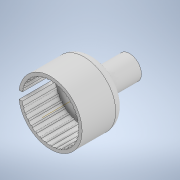
# Autodesk Inventor part: Coupler2
Saved by Autodesk Inventor 2020 (Build 240168000, 168)
## iProperties
Created: 2020-06-07
Part Number: Coupler2
Material: Generic
Document SubType Name: Modeling
Designer: Brandon
Density: 1 g/cm^3
Appearance: Default
Author: Brandon
Autodesk Inventor part; units mm, degrees
ref_plane "YZ Plane" through (0, 0, 0) normal (1, 0, 0) x (0, 1, 0)
ref_plane "XZ Plane" through (0, 0, 0) normal (0, 1, 0) x (-1, 0, 0)
ref_plane "XY Plane" through (0, 0, 0) normal (0, 0, 1) x (1, 0, 0)
sketch "Sketch1" plane through (0, 0, 0) normal (0, 0, 1) x (1, 0, 0)
  circle A0 centre (0, 0) radius 10.16
  dimension "d0" = 20.32
  constraints: 1 centre point, 1 coincident
  measures "d0" diameter of A0
extrude "Extrusion1" add sketch "Sketch1" against normal blind 25.4
sketch "Sketch2" plane through (0, 0, 0) normal (0, 0, 1) x (1, 0, 0)
  circle A0 centre (0, 0) radius 9.144
  dimension "d3" = 18.288
  constraints: 1 centre point, 1 coincident
  measures "d3" diameter of A0
extrude "Extrusion2" cut sketch "Sketch2" against normal blind 10.668
sketch "Sketch3" plane through (0, 0, -25.4) normal (0, 0, -1) x (-1, 0, 0)
  circle A0 centre (0, 0) radius 2.667
  line L0 (2.159, 1.5658) -> (2.159, -1.5658)
  dimension "d6" = 5.334
  dimension "d7" = 4.826
  constraints: 2 end point, 2 point on circle, 1 centre point, 1 coincident, 1 vertical
  measures "d6" diameter of A0
extrude "Extrusion3" cut sketch "Sketch3" against normal blind 11.43 contours L0 A0 picked at (-0.0356, -0.8771)
sketch "Sketch4" plane through (0, 0, -25.4) normal (0, 0, -1) x (-1, 0, 0)
  circle A0 centre (0, 0) radius 3.81
  circle A1 centre (0, 0) radius 10.16
  dimension "d10" = 7.62
  constraints: 2 centre point, 2 coincident
  measures "d10" diameter of A0
extrude "Extrusion4" cut sketch "Sketch4" against normal blind 11.43
fillet "Fillet2" radius 3.175 1 edges at (-10.16, 0, -13.97)
sketch "Sketch6" plane through (0, 0, 0) normal (0, 0, 1) x (1, 0, 0)
  line L0 (-10.922, -1.27) -> (-5.08, -1.27)
  line L1 (-5.08, -1.27) -> (-5.08, 1.27)
  line L2 (-5.08, 1.27) -> (-10.922, 1.27)
  line L3 (-10.922, 1.27) -> (-10.922, -1.27)
  point P0 (0, 0)
  dimension "d19" = 2.54
  dimension "d20" = 5.08
  dimension "d21" = 1.27
  constraints: 8 end point, 2 parallel, 1 horizontal, 1 perpendicular
  measures "d19" distance of L2.end L0.start
  measures "d20" distance from line of point (0, 0) L1
  measures "d21" distance from line of point (0, 0) L2
extrude "Extrusion6" cut sketch "Sketch6" against normal blind 10.668
sketch "Sketch7" plane through (0, 0, 0) normal (0, 0, 1) x (1, 0, 0)
  arc A0 (-9.0554, -1.27) -> (-9.0554, 1.27) centre (0, 0) ccw projected
  circle A1 centre (0, -9.144) radius 0.254
  dimension "d24" = 0.508
  constraints: 1 centre point, 1 point on circle
  measures "d24" diameter of A1
extrude "Extrusion7" add sketch "Sketch7" against normal blind 10.668
pattern_circular "Circular Pattern1" count 35 over 360 about axis through (0, 0, 0) along (0, 0, -1) of "Extrusion7"
sketch "Sketch8" plane through (0, 0, 0) normal (0, 0, 1) x (1, 0, 0)
  line L0 (-10.7775, -1.27) -> (-8.1519, -1.27)
  line L1 (-8.1519, -1.27) -> (-8.1519, 1.2704)
  line L2 (-8.1519, 1.2704) -> (-10.7775, 1.2704)
  line L3 (-10.7775, 1.2704) -> (-10.7775, -1.27)
  point P0 (0, 0)
  constraints: 8 end point, 2 parallel, 1 horizontal, 1 perpendicular
extrude "Extrusion8" cut sketch "Sketch8" against normal blind 10.668
sketch "Sketch9" plane through (0, 0, 0) normal (0, 0, 1) x (1, 0, 0)
  circle A0 centre (0, 0) radius 9.144
  line L0 (-9.2823, -1.8753) -> (-8.4046, -1.8753)
  line L1 (-8.4046, -1.8753) -> (-8.4046, -0.367)
  line L2 (-8.4046, -0.367) -> (-9.2823, -0.367)
  line L3 (-9.2823, -0.367) -> (-9.2823, -1.8753)
  point P0 (-9.1366, -0.367)
  point P1 (-8.9496, -1.8753)
  constraints: 8 end point, 2 parallel, 1 centre point, 1 coincident, 1 horizontal, 1 perpendicular
extrude "Extrusion9" cut sketch "Sketch9" against normal blind 10.668 contours L2 L1 L0 A0 picked at (-8.6163, -1.2062)
body "Solid1"
